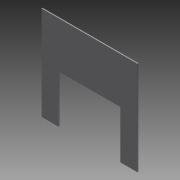
# Autodesk Inventor part: electrical board seal front
Saved by Autodesk Inventor 2012 (Build 160160000, 160)
## iProperties
Created: 2011-12-02
Part Number: electrical board seal front
Material: ABS Plastic
Document SubType Name: Modeling
Designer: Antonella
Mass: 638.358 g
Surface Area: 7626.19 cm^2
Volume: 602.225 cm^3
Density: 1.06 g/cm^3
Author: Antonella
Autodesk Inventor part; units mm, degrees
ref_plane "YZ Plane" through (0, 0, 0) normal (1, 0, 0) x (0, 1, 0)
ref_plane "XZ Plane" through (0, 0, 0) normal (0, 1, 0) x (-1, 0, 0)
sketch "Sketch1" plane through (0, 0, 0) normal (0, 0, 1) x (1, 0, 0)
  line L0 (-426.72, 0) -> (426.72, 0) projected
  line L1 (0, -417.83) -> (0, 417.83) projected
  line L2 (-304.8, 298.45) -> (304.8, 298.45)
  line L3 (304.8, 298.45) -> (304.8, -298.45)
  line L4 (304.8, -298.45) -> (-304.8, -298.45)
  line L5 (-304.8, -298.45) -> (-304.8, 298.45)
  point P0 (0, 0)
  point P1 (-304.8, 0)
  point P2 (0, 298.45)
  dimension "d0" = 609.6
  dimension "d1" = 596.9
  constraints: 8 end point, 2 midpoint, 2 parallel, 1 horizontal, 1 horizontal alignment, 1 perpendicular, 1 vertical alignment
  measures "d0" distance of L2.start L2.end
  measures "d1" distance of L4.end L2.start
extrude "Base" add sketch "Sketch1" along normal mid plane 6.35
sketch "Sketch2" plane through (0, 0, 3.175) normal (0, 0, 1) x (1, 0, 0)
  line L0 (304.8, -298.45) -> (-304.8, -298.45) projected
  line L1 (-196.85, -298.45) -> (-196.85, 6.35)
  line L2 (-196.85, 6.35) -> (196.85, 6.35)
  line L3 (196.85, 6.35) -> (196.85, -298.45)
  point P0 (0, 0)
  point P1 (0, 6.35)
  dimension "d4" = 304.8
  dimension "d5" = 393.7
  constraints: 6 end point, 3 perpendicular, 2 point on line, 1 midpoint, 1 vertical alignment
  measures "d4" distance between parallel lines of L0 L2
  measures "d5" distance of L1.end L2.end
extrude "Extrusion2" cut sketch "Sketch2" against normal through all
ref_plane "Work Plane1" through (-304.8, 152.4, 3.175) normal (0, 1, 0) x (1, 0, 0)
body "Solid1"
